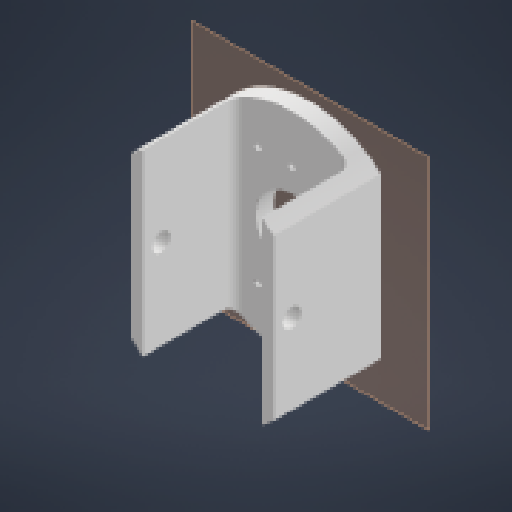
# Autodesk Inventor part: Part1
Saved by Autodesk Inventor 2023 (Build 270158000, 158)
## iProperties
Created: 2023-09-09
Part Number: Part1
Material: Generic
Document SubType Name: Modeling
Designer: philo
Density: 1 g/cm^3
Appearance: Default
Author: philo
Autodesk Inventor part; units mm, degrees
ref_plane "YZ Plane" through (0, 0, 0) normal (1, 0, 0) x (0, 1, 0)
ref_plane "XZ Plane" through (0, 0, 0) normal (0, 1, 0) x (-1, 0, 0)
ref_plane "XY Plane" through (0, 0, 0) normal (0, 0, 1) x (1, 0, 0)
ref_plane "Work Plane1" through (0, 0, 0) normal (0, 0, 1) x (1, 0, 0)
sketch "Sketch1" plane through (0, 0, 0) normal (0, 0, 1) x (1, 0, 0)
  circle A0 centre (-19, 33) radius 1.5 projected
  circle A1 centre (19, -33) radius 1.5 projected
  circle A2 centre (0, 33) radius 1.5 projected
  circle A3 centre (-19, -33) radius 1.5 projected
  circle A4 centre (0, -33) radius 1.5 projected
  circle A5 centre (19, 33) radius 1.5 projected
  circle A6 centre (0, 0) radius 60 projected
  circle A7 centre (8.9057, -8.0429) radius 1.5 projected
  circle A8 centre (8.0429, 8.9057) radius 1.5 projected
  circle A9 centre (-8.0429, -8.9057) radius 1.5 projected
  circle A10 centre (-8.9057, 8.0429) radius 1.5 projected
  circle A11 centre (0, 0) radius 4 projected
  circle A12 centre (-36.9264, 33.7112) radius 1.5 projected
  circle A13 centre (36.9264, -33.7112) radius 1.5 projected
  circle A14 centre (33.7112, 36.9264) radius 1.5 projected
  circle A15 centre (-33.7112, -36.9264) radius 1.5 projected
  line L0 (-40, -63) -> (40, -63)
  line L1 (40, -63) -> (40, 67)
  line L2 (40, 67) -> (-40, 67)
  line L3 (-40, 67) -> (-40, -63)
  point P0 (0, 0)
  point P1 (-40, 44.7214)
  point P2 (-40, -44.7214)
  point P3 (40, -44.7214)
  point P4 (40, 44.7214)
  dimension "d0" = 40
  dimension "d1" = 40
  dimension "d2" = 130
  dimension "d3" = 67
  constraints: 8 end point, 2 parallel, 1 horizontal, 1 perpendicular
  measures "d0" distance from line of L3 point (0, 0)
  measures "d1" distance from line of point (0, 0) L1
  measures "d2" distance between parallel lines of L0 L2
  measures "d3" distance from line of L2 point (0, 0)
extrude "Extrusion1" add sketch "Sketch1" along normal blind 10 contours L1 A6 L3 | A12 | A13 | A14 | A15
sketch "Sketch2" plane through (0, 0, 10) normal (0, 0, 1) x (1, 0, 0)
  circle A0 centre (0, 0) radius 20
  dimension "d6" = 40
  constraints: 1 centre point, 1 coincident
  measures "d6" diameter of A0
extrude "Extrusion2" cut sketch "Sketch2" against normal blind 10
sketch "Sketch3" plane through (0, 0, 10) normal (0, 0, 1) x (1, 0, 0)
  circle A0 centre (0, 0) radius 20 projected
  arc A1 (-40, -44.7214) -> (40, -44.7214) centre (0, 0) ccw projected
  line L0 (40, -44.7214) -> (40, 44.7214) projected
  arc A2 (40, 44.7214) -> (-40, 44.7214) centre (0, 0) ccw projected
  line L1 (-40, 44.7214) -> (-40, -44.7214) projected
  circle A3 centre (19, 33) radius 1.5 projected
  circle A4 centre (0, -33) radius 1.5 projected
  circle A5 centre (-19, -33) radius 1.5 projected
  circle A6 centre (0, 33) radius 1.5 projected
  circle A7 centre (19, -33) radius 1.5 projected
  circle A8 centre (-19, 33) radius 1.5 projected
  line L2 (-40, -57.711) -> (-33, -57.711)
  line L3 (-33, -57.711) -> (-33, 58.4565)
  line L4 (-33, 58.4565) -> (-40, 58.4565)
  line L5 (-40, 58.4565) -> (-40, -57.711)
  line L6 (40, -61.1567) -> (33, -61.1567)
  line L7 (33, -61.1567) -> (33, 64.5274)
  line L8 (33, 64.5274) -> (40, 64.5274)
  line L9 (40, 64.5274) -> (40, -61.1567)
  point P0 (33, 50.1099)
  point P1 (33, -50.1099)
  point P2 (-33, -50.1099)
  point P3 (-33, 50.1099)
  dimension "d9" = 7
  dimension "d10" = 7
  constraints: 16 end point, 4 parallel, 2 horizontal, 2 perpendicular, 1 point on line
  measures "d9" distance of L4.end L3.end
  measures "d10" distance of L7.end L8.end
extrude "Extrusion3" add sketch "Sketch3" along normal blind 50 contours L1 A2 L3 A1 | L7 A2 L0 A1
fillet "Fillet1" radius 5 2 edges at (-33, 0, 10) (33, 0, 10)
sketch "Sketch4" plane through (40, -44.7214, 0) normal (1, 0, 0) x (0, 0, -1)
  circle A0 centre (-50, 44.8312) radius 5
  line L0 (-60, 0) -> (-60, 89.4427) projected
  line L1 (-15, 94.8312) -> (-60, 94.8312) projected
  point P0 (0, 44.7214)
  dimension "d14" = 10
  dimension "d15" = 10
  dimension "d16" = 50
  constraints: 1 centre point
  measures "d14" diameter of A0
  measures "d15" distance from line of L0 A0.centre
  measures "d16" distance from line of L1 A0.centre
extrude "Extrusion4" cut sketch "Sketch4" against normal blind 200
body "Solid1"
